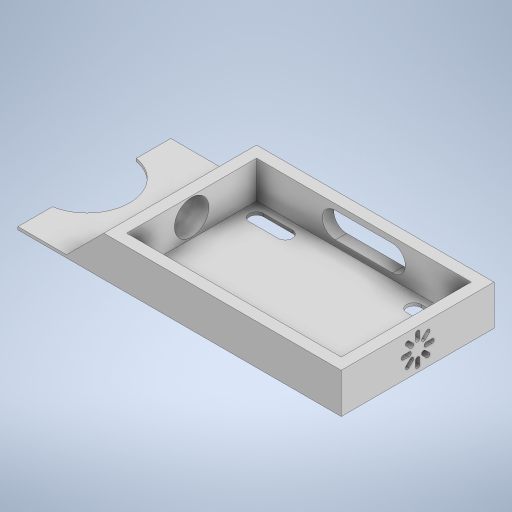
# Autodesk Inventor part: klp
Saved by Autodesk Inventor 2024.3 (Build 283343000, 343)
## iProperties
Created: 2024-08-13
Part Number: klp
Material: Ogólny
Document SubType Name: Modeling
Designer: User
Density: 1 g/cm^3
Appearance: Domyślna
Author: User
Autodesk Inventor part; units mm, degrees
ref_plane "YZ Plane" through (0, 0, 0) normal (1, 0, 0) x (0, 1, 0)
ref_plane "XZ Plane" through (0, 0, 0) normal (0, 1, 0) x (-1, 0, 0)
ref_plane "XY Plane" through (0, 0, 0) normal (0, 0, 1) x (1, 0, 0)
sketch "Szkic1" plane through (0, 0, 0) normal (0, 1, 0) x (-1, 0, 0)
  line L0 (0, 0) -> (0, -53.4)
  line L1 (0, -53.4) -> (113, -53.4)
  line L2 (0, -53.4) -> (113, -53.4) construction
  line L3 (0, -53.4) -> (113, -53.4)
  line L4 (113, -53.4) -> (113, 0)
  line L5 (113, 0) -> (0, 0)
  line L6 (0, 0) -> (0, -53.4)
  dimension "d0" = 53.4
  dimension "d1" = 113
  dimension "d2" = 0
  constraints: 14 end point, 3 horizontal, 2 parallel, 1 collinear, 1 perpendicular, 1 vertical
  measures "d0" distance of L0.start L0.end
  measures "d1" distance of L0.end L1.end
  measures "d2" distance between parallel lines of L1 L2
extrude "Wyciągnięcie proste1" add sketch "Szkic1" along normal blind 1
sketch "Szkic2" plane through (0, 1, 0) normal (0, 1, 0) x (1, 0, 0)
  line L0 (-113, 53.4) -> (-113, 0) projected
  line L1 (-113, 0) -> (-83, 0)
  line L2 (-113, 0) -> (0, 0) projected
  line L3 (-83, 0) -> (-83, 53.4)
  line L4 (0, 53.4) -> (-113, 53.4) projected
  line L5 (-83, 0) -> (0, 0)
  line L6 (0, 0) -> (0, 53.4)
  line L7 (0, 53.4) -> (-83, 53.4)
  line L8 (-83, 53.4) -> (-83, 0)
  line L9 (-83, 0) -> (-79, 0)
  line L10 (-79, 0) -> (-79, 4)
  line L11 (0, 53.4) -> (-4, 53.4)
  line L12 (-4, 53.4) -> (-4, 49.4)
  line L13 (-79, 4) -> (-4, 4)
  line L14 (-4, 4) -> (-4, 49.4)
  line L15 (-4, 49.4) -> (-79, 49.4)
  line L16 (-79, 49.4) -> (-79, 4)
  dimension "d5" = 30
  dimension "d6" = 4
  dimension "d7" = 4
  dimension "d8" = 4
  dimension "d9" = 4
  constraints: 28 end point, 5 perpendicular, 4 parallel, 4 point on line, 2 horizontal
  measures "d5" distance of L0.end L1.end
  measures "d6" distance of L1.end L9.end
  measures "d7" distance of L9.end L10.end
  measures "d8" distance of L4.start L11.end
  measures "d9" distance of L11.end L12.end
extrude "Wyciągnięcie proste2" add sketch "Szkic2" along normal blind 13 contours L4 L12 L15 L16 L10 L2 L3 | L4 L6 L2 L10 L13 L14 L12
sketch "Szkic3" plane through (0, 1, 0) normal (0, 1, 0) x (1, 0, 0)
  line L0 (-113, 53.4) -> (-113, 0) projected
  line L1 (-113, 26.7) -> (-113, 12.05)
  line L2 (-113, 26.7) -> (-113, 41.35)
  arc A0 (-113, 12.05) -> (-113, 41.35) centre (-115.5542, 26.7) ccw
  point P0 (0, 0)
  dimension "d12" = 14.65
  dimension "d13" = 14.65
  dimension "d14" = 14.871
  constraints: 4 end point, 2 point on circle, 2 point on line, 1 centre point, 1 midpoint
  measures "d12" distance of L1.start L1.end
  measures "d13" distance of L1.start L2.end
  measures "d14" radius of A0
extrude "Wyciągnięcie proste3" cut sketch "Szkic3" against normal blind 13
chamfer "Faza1" distance 13 angle 45 1 edges at (-83, 1, -26.7)
sketch "Szkic4" plane through (-79, 1, -4) normal (1, 0, 0) x (0, 0, -1)
  line L0 (45.4, 0) -> (0, 0) projected
  line L1 (22.7, 0) -> (22.7, 13)
  line L2 (0, 13) -> (45.4, 13) projected
  circle A0 centre (22.7, 6.5) radius 6
  point P0 (-4, -1)
  dimension "d20" = 12
  constraints: 3 midpoint, 2 end point, 1 centre point
  measures "d20" diameter of A0
extrude "Wyciągnięcie proste4" cut sketch "Szkic4" against normal through all
sketch "Szkic5" plane through (0, 0, 0) normal (1, 0, 0) x (0, 0, -1)
  line L0 (0, 0) -> (0, 14) projected
  line L1 (0, 7) -> (53.4, 7)
  line L2 (53.4, 0) -> (53.4, 14) projected
  line L3 (4, 14) -> (49.4, 14) projected
  line L4 (26.7, 14) -> (26.7, 0)
  line L5 (0, 0) -> (53.4, 0) projected
  circle A0 centre (26.7, 7) radius 2
  line L6 (26.7, 9) -> (26.7, 10)
  line L7 (26.7, 10) -> (26.7, 12) construction
  line L8 (27.45, 10) -> (27.45, 12)
  line L9 (25.95, 12) -> (25.95, 10)
  arc A1 (25.95, 10) -> (27.45, 10) centre (26.7, 10) ccw
  arc A2 (27.45, 12) -> (25.95, 12) centre (26.7, 12) ccw
  line L10 (28.1142, 8.4142) -> (28.8213, 9.1213)
  line L11 (28.8213, 9.1213) -> (30.2355, 10.5355) construction
  line L12 (29.7052, 11.0659) -> (28.291, 9.6517)
  arc A3 (28.291, 9.6517) -> (29.3517, 8.591) centre (28.8213, 9.1213) ccw
  arc A4 (30.7659, 10.0052) -> (29.7052, 11.0659) centre (30.2355, 10.5355) ccw
  line L13 (29.3517, 8.591) -> (30.7659, 10.0052)
  line L14 (28.7, 7) -> (29.7, 7)
  line L15 (29.7, 7) -> (31.7, 7) construction
  line L16 (31.7, 7.75) -> (29.7, 7.75)
  arc A5 (29.7, 7.75) -> (29.7, 6.25) centre (29.7, 7) ccw
  arc A6 (31.7, 6.25) -> (31.7, 7.75) centre (31.7, 7) ccw
  line L17 (29.7, 6.25) -> (31.7, 6.25)
  line L18 (28.1142, 5.5858) -> (28.8213, 4.8787)
  line L19 (28.8213, 4.8787) -> (30.2355, 3.4645) construction
  line L20 (30.7659, 3.9948) -> (29.3517, 5.409)
  arc A7 (29.3517, 5.409) -> (28.291, 4.3483) centre (28.8213, 4.8787) ccw
  arc A8 (29.7052, 2.9341) -> (30.7659, 3.9948) centre (30.2355, 3.4645) ccw
  line L21 (28.291, 4.3483) -> (29.7052, 2.9341)
  line L22 (26.7, 5) -> (26.7, 4)
  line L23 (26.7, 4) -> (26.7, 2) construction
  line L24 (27.45, 2) -> (27.45, 4)
  arc A9 (27.45, 4) -> (25.95, 4) centre (26.7, 4) ccw
  arc A10 (25.95, 2) -> (27.45, 2) centre (26.7, 2) ccw
  line L25 (25.95, 4) -> (25.95, 2)
  line L26 (25.2858, 5.5858) -> (24.5787, 4.8787)
  line L27 (24.5787, 4.8787) -> (23.1645, 3.4645) construction
  line L28 (23.6948, 2.9341) -> (25.109, 4.3483)
  arc A11 (25.109, 4.3483) -> (24.0483, 5.409) centre (24.5787, 4.8787) ccw
  arc A12 (22.6341, 3.9948) -> (23.6948, 2.9341) centre (23.1645, 3.4645) ccw
  line L29 (24.0483, 5.409) -> (22.6341, 3.9948)
  line L30 (24.7, 7) -> (23.7, 7)
  line L31 (23.7, 7) -> (21.7, 7) construction
  line L32 (21.7, 6.25) -> (23.7, 6.25)
  arc A13 (23.7, 6.25) -> (23.7, 7.75) centre (23.7, 7) ccw
  arc A14 (21.7, 7.75) -> (21.7, 6.25) centre (21.7, 7) ccw
  line L33 (23.7, 7.75) -> (21.7, 7.75)
  line L34 (25.2858, 8.4142) -> (24.5787, 9.1213)
  line L35 (24.5787, 9.1213) -> (23.1645, 10.5355) construction
  line L36 (22.6341, 10.0052) -> (24.0483, 8.591)
  arc A15 (24.0483, 8.591) -> (25.109, 9.6517) centre (24.5787, 9.1213) ccw
  arc A16 (23.6948, 11.0659) -> (22.6341, 10.0052) centre (23.1645, 10.5355) ccw
  line L37 (25.109, 9.6517) -> (23.6948, 11.0659)
  point P0 (26.7, 11)
  point P1 (29.5284, 9.8284)
  point P2 (30.7, 7)
  point P3 (29.5284, 4.1716)
  point P4 (26.7, 3)
  point P5 (23.8716, 4.1716)
  point P6 (22.7, 7)
  point P7 (23.8716, 9.8284)
  dimension "d23" = 4
  dimension "d24" = 1
  dimension "d25" = 2
  dimension "d26" = 1.5
  dimension "d29" = 360
  constraints: 84 end point, 32 point on circle, 16 centre point, 6 midpoint, 4 tangent, 3 point on line, 1 parallel, 1 vertical alignment, 115 other
  measures "d24" distance of L6.start L6.end
  measures "d25" distance of L6.end L7.end
  measures "d26" diameter of A2
extrude "Wyciągnięcie proste5" cut sketch "Szkic5" against normal blind 10 contours A15 L36 A16 L37 | A1 L9 A2 L4 | L4 A2 L8 A1 | A3 L12 A4 L13 | A11 L28 A12 L29 | A7 L20 A8 L21 | A14 L33 A13 L1 | L1 A13 L32 A14 | A10 L25 A9 L4 | L4 A9 L24 A10 | A6 L17 A5 L1 | L1 A5 L16 A6
sketch "Szkic6" plane through (0, 1, 0) normal (0, 1, 0) x (1, 0, 0)
  line L0 (-4, 4) -> (-4, 49.4) projected
  line L1 (-4, 4) -> (-4, 9)
  line L2 (-4, 9) -> (-9, 9)
  line L3 (-9, 9) -> (-19, 9) construction
  line L4 (-9, 11.5) -> (-19, 11.5)
  line L5 (-19, 6.5) -> (-9, 6.5)
  arc A0 (-9, 6.5) -> (-9, 11.5) centre (-9, 9) ccw
  arc A1 (-19, 11.5) -> (-19, 6.5) centre (-19, 9) ccw
  line L6 (-4, 26.7) -> (-79, 26.7)
  line L7 (-79, 49.4) -> (-79, 4) projected
  line L8 (-79, 4) -> (-4, 4) projected
  line L9 (-41.5, 4) -> (-41.5, 49.4)
  line L10 (-4, 49.4) -> (-79, 49.4) projected
  line L11 (-74, 9) -> (-64, 9) construction
  line L12 (-74, 11.5) -> (-64, 11.5)
  line L13 (-64, 6.5) -> (-74, 6.5)
  arc A2 (-74, 11.5) -> (-74, 6.5) centre (-74, 9) ccw
  arc A3 (-64, 6.5) -> (-64, 11.5) centre (-64, 9) ccw
  line L14 (-4, 44.4) -> (-9, 44.4)
  line L15 (-9, 44.4) -> (-19, 44.4) construction
  line L16 (-9, 41.9) -> (-19, 41.9)
  line L17 (-19, 46.9) -> (-9, 46.9)
  arc A4 (-9, 41.9) -> (-9, 46.9) centre (-9, 44.4) ccw
  arc A5 (-19, 46.9) -> (-19, 41.9) centre (-19, 44.4) ccw
  line L18 (-41.5, 49.4) -> (-41.5, 4)
  arc A6 (-74, 46.9) -> (-74, 41.9) centre (-74, 44.4) ccw
  line L19 (-74, 44.4) -> (-64, 44.4) construction
  line L20 (-64, 46.9) -> (-74, 46.9)
  line L21 (-74, 41.9) -> (-64, 41.9)
  arc A7 (-64, 41.9) -> (-64, 46.9) centre (-64, 44.4) ccw
  point P0 (0, 0)
  point P1 (-14, 9)
  point P2 (-69, 9)
  point P3 (-14, 44.4)
  point P4 (-69, 44.4)
  dimension "d33" = 5
  dimension "d34" = 5
  dimension "d35" = 10
  dimension "d36" = 5
  constraints: 44 end point, 24 symmetric about line, 16 point on circle, 8 centre point, 5 midpoint, 4 tangent, 1 horizontal, 1 parallel, 1 perpendicular, 1 point on line, 6 other
  measures "d33" distance of L0.start L1.end
  measures "d34" distance of L1.end L2.end
  measures "d35" distance of L2.end L3.end
  measures "d36" diameter of A1
extrude "Wyciągnięcie proste6" cut sketch "Szkic6" against normal blind 10 contours A0 L5 A1 L4 | A4 L16 A5 L17 | L12 A3 L13 A2 | L20 A7 L21 A6
sketch "Szkic7" plane through (0, 0, -53.4) normal (0, 0, -1) x (-1, 0, 0)
  line L0 (79, 1) -> (4, 1) projected
  line L1 (41.5, 1) -> (41.5, 14)
  line L2 (4, 14) -> (79, 14) projected
  line L3 (79, 1.5) -> (79, 13.5) projected
  line L4 (79, 7.5) -> (41.5, 7.5)
  line L5 (41.5, 7.5) -> (31.5, 7.5)
  line L6 (31.5, 7.5) -> (51.5, 7.5) construction
  line L7 (31.5, 3) -> (51.5, 3)
  line L8 (51.5, 12) -> (31.5, 12)
  arc A0 (31.5, 12) -> (31.5, 3) centre (31.5, 7.5) ccw
  arc A1 (51.5, 3) -> (51.5, 12) centre (51.5, 7.5) ccw
  point P0 (0, 0)
  dimension "d39" = 10
  dimension "d40" = 20
  dimension "d41" = 9
  constraints: 14 end point, 5 midpoint, 4 point on circle, 4 tangent, 2 centre point, 2 point on line, 1 parallel
  measures "d39" distance of L4.end L5.end
  measures "d40" distance of L5.end L6.end
  measures "d41" diameter of A1
extrude "Wyciągnięcie proste7" cut sketch "Szkic7" against normal blind 10
